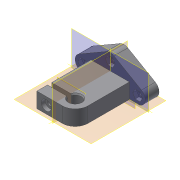
# Autodesk Inventor part: Cycl_soporteYfrenteDerecha
Saved by Autodesk Inventor 2015 SP2 (Build 190223200, 223)
## iProperties
Created: 2015-05-04
Material: Genérico
Document SubType Name: Modeling
Designer: E.Beroiz
Density: 1 g/cm^3
Appearance: Valor por defecto
Description: Cycl_soporteYfrenteDerecha
Author: E.Beroiz
Autodesk Inventor part; units mm, degrees
sketch "Boceto1" plane through (0, 0, 0) normal (0, 0, 1) x (1, 0, 0)
  line L0 (-13.875, 0) -> (13.875, 0)
  line L1 (13.875, 0) -> (13.875, -39.25)
  line L2 (13.875, -39.25) -> (-13.875, -39.25)
  line L3 (-13.875, -39.25) -> (-13.875, 0)
  point P0 (0, 0)
  point P1 (0, 0)
  dimension "d0" = 27.75
  dimension "d1" = 39.25
  constraints: 8 end point, 2 coincident, 2 parallel, 1 horizontal, 1 midpoint, 1 perpendicular
  measures "d0" distance of L1.end L2.end
  measures "d1" distance of L0.end L1.end
extrude "Extrusión1" add sketch "Boceto1" along normal blind 11
fillet "Empalme1" radius 9.25 1 edges at (13.875, -39.25, 5.5)
sketch "Boceto2" plane through (0, 0, 11) normal (0, 0, 1) x (1, 0, 0)
  arc A0 (4.625, -39.25) -> (13.875, -30) centre (4.625, -30) ccw projected
  line L0 (13.875, -30) -> (13.875, 0) projected
  line L1 (13.875, 0) -> (-13.875, 0) projected
  line L2 (-13.875, 0) -> (-13.875, -39.25) projected
  line L3 (-13.875, -39.25) -> (4.625, -39.25) projected
  line L4 (-13.875, 0) -> (-13.875, -39.25) projected
  line L5 (-13.875, -31.5) -> (0.4886, -31.5)
  line L6 (-13.875, -28.5) -> (0.4886, -28.5)
  arc A1 (0.4886, -31.5) -> (0.4886, -28.5) centre (4.625, -30) ccw
  point P0 (0, 0)
  dimension "d5" = 3
  dimension "d6" = 7.75
  dimension "d13" = 1.5
  dimension "d62" = 4.4
  dimension "d63" = 9.25
  constraints: 4 end point, 2 point on circle, 2 point on line, 1 centre point, 1 horizontal, 1 perpendicular
  measures "d5" distance between parallel lines of L6 L5
  measures "d6" distance between parallel lines of L3 L5
  measures "d13" distance from line of L5 A1.centre
  measures "d62" radius of A1
  measures "d63" distance from line of A0.centre L0
extrude "Extrusión2" cut sketch "Boceto2" against normal blind 11 contours L2 L6 A1 L5
sketch "Boceto3" plane through (0, 0, 0) normal (0, 1, 0) x (-1, 0, 0)
  line L0 (-19.875, 0) -> (19.875, 0)
  line L1 (22.6302, 10.2645) -> (2.7552, 21.7625)
  line L2 (-2.7552, 21.7625) -> (-22.6302, 10.2645)
  line L3 (13.875, 0) -> (-13.875, 0) projected
  arc A0 (-22.6302, 10.2645) -> (-19.875, 0) centre (-19.875, 5.502) ccw
  arc A1 (19.875, 0) -> (22.6302, 10.2645) centre (19.875, 5.502) ccw
  arc A2 (2.7552, 21.7625) -> (-2.7552, 21.7625) centre (0, 17) ccw
  point P0 (0, 0)
  point P1 (0, 23.3564)
  point P2 (0, 0)
  point P3 (0, 0)
  point P4 (0, 0)
  point P5 (0, 0)
  dimension "d21" = 30.05
  dimension "d23" = 39.75
  dimension "d25" = 17
  constraints: 6 end point, 6 point on circle, 6 tangent, 4 midpoint, 3 centre point, 2 equal radius, 2 point on line, 2 vertical alignment, 1 coincident, 1 equal length, 1 horizontal, 1 horizontal alignment
  measures "d21" angle of L0 L1
  measures "d23" distance of A1.centre A0.centre
  measures "d25" distance from line of L0 A2.centre
extrude "Extrusión3" add sketch "Boceto3" along normal blind 10
ref_plane "Plano de trabajo2" through (0, 7.2, 0) normal (0, 1, 0) x (1, 0, 0)
sketch "Boceto5" plane through (0, 7.2, 0) normal (0, 1, 0) x (1, 0, 0)
  line L0 (19.875, 0) -> (-19.875, 0) projected
  arc A0 (-19.875, 0) -> (-22.6302, -10.2645) centre (-19.875, -5.502) ccw projected
  line L1 (-22.6302, -10.2645) -> (-2.7552, -21.7625) projected
  arc A1 (-2.7552, -21.7625) -> (2.7552, -21.7625) centre (0, -17) ccw projected
  line L2 (2.7552, -21.7625) -> (22.6302, -10.2645) projected
  arc A2 (22.6302, -10.2645) -> (19.875, 0) centre (19.875, -5.502) ccw projected
  circle A3 centre (19.875, -5.502) radius 1.875
  circle A4 centre (0, -17) radius 1.875
  circle A5 centre (-19.875, -5.502) radius 1.875
  point P0 (0, 0)
  dimension "d33" = 3.75
  dimension "d34" = 3.75
  dimension "d35" = 3.75
  constraints: 3 centre point, 3 coincident
  measures "d33" diameter of A3
  measures "d34" diameter of A4
  measures "d35" diameter of A5
extrude "Extrusión5" cut sketch "Boceto5" along normal through all both and the other way through all contours A3 | A4 | A5
sketch "Boceto6" plane through (0, 0, 0) normal (0, -1, 0) x (1, 0, 0)
  circle A0 centre (0, 17) radius 1.875 projected
  circle A1 centre (19.875, 5.502) radius 1.875 projected
  circle A2 centre (-19.875, 5.502) radius 1.875 projected
  line L0 (13.875, 0) -> (13.875, 11) projected
  line L1 (19.875, 0) -> (13.875, 0) projected
  arc A3 (19.875, 0) -> (22.6302, 10.2645) centre (19.875, 5.502) ccw projected
  line L2 (2.7552, 21.7625) -> (22.6302, 10.2645) projected
  arc A4 (2.7552, 21.7625) -> (-2.7552, 21.7625) centre (0, 17) ccw projected
  line L3 (-22.6302, 10.2645) -> (-2.7552, 21.7625) projected
  arc A5 (-22.6302, 10.2645) -> (-19.875, 0) centre (-19.875, 5.502) ccw projected
  line L4 (-13.875, 0) -> (-19.875, 0) projected
  line L5 (-13.875, 0) -> (-13.875, 11) projected
  line L6 (13.875, 11) -> (-13.875, 11) projected
  line L7 (-18.0852, 8.602) -> (-16.2954, 5.502)
  line L8 (-16.2954, 5.502) -> (-18.0852, 2.402)
  line L9 (-18.0852, 2.402) -> (-21.6648, 2.402)
  line L10 (-21.6648, 2.402) -> (-23.4546, 5.502)
  line L11 (-23.4546, 5.502) -> (-21.6648, 8.602)
  line L12 (-21.6648, 8.602) -> (-18.0852, 8.602)
  line L13 (1.7898, 20.1) -> (3.5796, 17)
  line L14 (3.5796, 17) -> (1.7898, 13.9)
  line L15 (1.7898, 13.9) -> (-1.7898, 13.9)
  line L16 (-1.7898, 13.9) -> (-3.5796, 17)
  line L17 (-3.5796, 17) -> (-1.7898, 20.1)
  line L18 (-1.7898, 20.1) -> (1.7898, 20.1)
  line L19 (18.0852, 8.602) -> (21.6648, 8.602)
  line L20 (21.6648, 8.602) -> (23.4546, 5.502)
  line L21 (23.4546, 5.502) -> (21.6648, 2.402)
  line L22 (21.6648, 2.402) -> (18.0852, 2.402)
  line L23 (18.0852, 2.402) -> (16.2954, 5.502)
  line L24 (16.2954, 5.502) -> (18.0852, 8.602)
  point P0 (0, 0)
  dimension "d38" = 6.2
  dimension "d39" = 6.2
  dimension "d40" = 6.2
  constraints: 36 end point, 3 coincident, 3 horizontal, 39 other
  measures "d38" distance between parallel lines of L15 L18
  measures "d39" distance between parallel lines of L22 L19
  measures "d40" distance between parallel lines of L9 L12
extrude "Extrusión6" cut sketch "Boceto6" against normal blind 2.8 contours L7 L8 L9 L10 L11 L12 | L13 L14 L15 L16 L17 L18 | L19 L20 L21 L22 L23 L24
sketch "Boceto7" plane through (-13.875, -39.25, 0) normal (0, -1, 0) x (1, 0, 0)
  circle A0 centre (6.8, 5.5) radius 3.6
  line L0 (18.5, 0) -> (0, 0) projected
  line L1 (0, 0) -> (0, 11) projected
  point P0 (13.875, 0)
  dimension "d43" = 7.2
  dimension "d44" = 5.5
  dimension "d45" = 6.8
  constraints: 1 centre point
  measures "d43" diameter of A0
  measures "d44" distance from line of L0 A0.centre
  measures "d45" distance from line of L1 A0.centre
extrude "Extrusión7" cut sketch "Boceto7" against normal blind 2.8
sketch "Boceto8" plane through (-7.075, -36.45, 5.5) normal (0, -1, 0) x (1, 0, 0)
  circle A0 centre (0, 0) radius 3.6 projected
  circle A1 centre (0, 0) radius 1.875
  point P0 (7.075, -5.5)
  dimension "d48" = 3.75
  constraints: 1 centre point, 1 coincident
  measures "d48" diameter of A1
extrude "Extrusión8" cut sketch "Boceto8" against normal blind 26.4 contours A1
ref_plane "Plano de trabajo3" through (-13.875, -23.54, 0) normal (0, -1, 0) x (1, 0, 0)
sketch "Boceto9" plane through (-13.875, -23.54, 0) normal (0, -1, 0) x (1, 0, 0)
  circle A0 centre (6.8, 5.5) radius 1.875 projected
  line L0 (27.75, 11) -> (0, 11) projected
  line L1 (0, 0) -> (0, 11) projected
  line L2 (-21.6528, 0) -> (49.4028, 0) projected
  line L3 (8.7816, 8.5126) -> (10.3998, 5.2902)
  line L4 (10.3998, 5.2902) -> (8.4182, 2.2776)
  line L5 (8.7816, 8.5126) -> (0, 8.5126)
  line L6 (8.4182, 2.2776) -> (0, 2.2776)
  point P0 (13.875, 0)
  dimension "d53" = 120
  dimension "d56" = 6.235
  dimension "d57" = 8.7816
  constraints: 8 end point, 2 perpendicular, 2 point on line, 1 coincident, 4 other
  measures "d53" angle of L4 L3
  measures "d56" distance between parallel lines of L6 L5
  measures "d57" distance of L5.end L3.start
extrude "Extrusión9" cut sketch "Boceto9" along normal mid plane 2.8
sketch "Boceto10" plane through (0, 0, 0) normal (0, 0, -1) x (-1, 0, 0)
  line L0 (-6.6202, -3.2438) -> (-7.3905, -2.9152) construction
  line L1 (-8.0553, -2.0944) -> (-6.2205, -2.0944) construction
  line L2 (-7.3905, -2.9152) -> (-8.2942, -2.6479) construction
  line L3 (-8.8708, -2.1991) -> (-8.0553, -2.0944) construction
  line L4 (-8.2942, -2.6479) -> (-9.3576, -2.433) construction
  line L5 (-9.521, -2.3562) -> (-8.8708, -2.1991) construction
  line L6 (-9.5623, -2.392) -> (-9.521, -2.3562) construction
  line L7 (-9.3576, -2.433) -> (-9.5623, -2.392) construction
  arc A0 (-6.6202, -3.2438) -> (-9.5623, -2.392) centre (-11.1752, -13.4701) ccw
  line L8 (-4.1904, -17.1175) -> (-4.9646, -16.4122) construction
  line L9 (-2.3638, -18.1479) -> (-2.8515, -17.944) construction
  line L10 (-2.2067, -18.1953) -> (-2.372, -18.0796) construction
  line L11 (-6.5651, -9.2139) -> (-6.3061, -8.5334) construction
  line L12 (-6.7552, -9.9275) -> (-6.5651, -9.2139) construction
  line L13 (-6.8626, -10.619) -> (-6.7552, -9.9275) construction
  line L14 (-6.3061, -8.5334) -> (-5.981, -7.886) construction
  line L15 (-5.981, -7.886) -> (-5.5953, -7.2826) construction
  line L16 (-5.5953, -7.2826) -> (-5.1545, -6.7234) construction
  line L17 (-4.6724, -6.0787) -> (-4.733, -5.5552) construction
  line L18 (-4.6614, -6.2109) -> (-4.6724, -6.0787) construction
  line L19 (-5.1545, -6.7234) -> (-4.6614, -6.2109) construction
  arc A1 (-4.6614, -6.2109) -> (-6.8626, -10.619) centre (0.1756, -11.3801) ccw
  line L20 (-6.8489, -12.3602) -> (-1.9257, -12.3602)
  line L21 (-2.0248, -10.619) -> (-6.8626, -10.619) construction
  line L22 (-2.0248, -10.619) -> (-6.8626, -10.619)
  line L23 (-3.3198, -17.7016) -> (-3.7661, -17.4261) construction
  line L24 (-3.7661, -17.4261) -> (-4.1904, -17.1175) construction
  line L25 (-2.8515, -17.944) -> (-3.3198, -17.7016) construction
  line L26 (-4.9646, -16.4122) -> (-5.6285, -15.594) construction
  line L27 (-5.6285, -15.594) -> (-5.9123, -15.1504) construction
  line L28 (-5.9123, -15.1504) -> (-6.1658, -14.682) construction
  arc A2 (-6.8489, -12.3602) -> (-2.3638, -18.1479) centre (0.1619, -11.559) ccw
  line L29 (-6.1658, -14.682) -> (-6.3834, -14.1944) construction
  line L30 (-0.5371, -13.4071) -> (-0.1239, -13.4484) construction
  line L31 (-0.9228, -13.2858) -> (-0.5371, -13.4071) construction
  line L32 (-1.2727, -13.0985) -> (-0.9228, -13.2858) construction
  line L33 (-6.8489, -12.3602) -> (-1.9257, -12.3602) construction
  line L34 (-6.3834, -14.1944) -> (-6.568, -13.6847) construction
  line L35 (-6.568, -13.6847) -> (-6.7112, -13.1613) construction
  line L36 (-6.7112, -13.1613) -> (-6.8268, -12.553) construction
  line L37 (-6.8268, -12.553) -> (-6.8489, -12.3602) construction
  line L38 (1.5815, -12.542) -> (1.7688, -12.1921) construction
  line L39 (1.025, -13.0985) -> (1.328, -12.845) construction
  line L40 (0.6751, -13.2858) -> (1.025, -13.0985) construction
  line L41 (0.2894, -13.4071) -> (0.6751, -13.2858) construction
  line L42 (-0.1239, -13.4484) -> (0.2894, -13.4071) construction
  line L43 (1.328, -12.845) -> (1.5815, -12.542) construction
  line L44 (1.328, -9.9412) -> (1.025, -9.6905) construction
  line L45 (1.025, -9.6905) -> (0.6751, -9.5004) construction
  line L46 (1.7688, -10.5942) -> (1.5815, -10.2443) construction
  line L47 (1.5815, -10.2443) -> (1.328, -9.9412) construction
  line L48 (1.89, -10.9799) -> (1.7688, -10.5942) construction
  line L49 (0.6751, -9.5004) -> (0.2894, -9.382) construction
  line L50 (1.9314, -11.3931) -> (1.89, -10.9799) construction
  line L51 (0.2894, -9.382) -> (-0.1239, -9.3406) construction
  line L52 (-1.9257, -12.3602) -> (-1.8292, -12.542) construction
  line L53 (-1.8292, -12.542) -> (-1.5758, -12.845) construction
  line L54 (-1.5758, -12.845) -> (-1.2727, -13.0985) construction
  line L55 (1.89, -11.8064) -> (1.9314, -11.3931) construction
  line L56 (1.7688, -12.1921) -> (1.89, -11.8064) construction
  arc A3 (-1.9257, -12.3602) -> (-2.0248, -10.619) centre (-0.0805, -11.3816) ccw
  line L57 (-2.6748, -2.6372) -> (-1.5397, -2.9457) construction
  arc A4 (2.4908, -4.8109) -> (-9.5623, -2.392) centre (-6.7465, -19.6002) ccw
  line L58 (-3.8457, -2.3892) -> (-2.6748, -2.6372) construction
  line L59 (-5.9617, -3.6405) -> (-6.6202, -3.2438) construction
  line L60 (-5.5678, -3.9821) -> (-5.9617, -3.6405) construction
  line L61 (-6.2205, -2.0944) -> (-5.0331, -2.2074) construction
  line L62 (-5.2317, -4.3596) -> (-5.5678, -3.9821) construction
  line L63 (-5.0002, -4.7342) -> (-5.2317, -4.3596) construction
  arc A5 (-4.6614, -6.2109) -> (-6.6202, -3.2438) centre (-7.8027, -6.1546) ccw
  line L64 (-4.8377, -5.1199) -> (-5.0002, -4.7342) construction
  line L65 (-4.733, -5.5552) -> (-4.8377, -5.1199) construction
  line L66 (-5.0331, -2.2074) -> (-3.8457, -2.3892) construction
  line L67 (1.477, -4.1745) -> (2.2925, -4.6676) construction
  line L68 (0.5541, -3.7199) -> (1.477, -4.1745) construction
  line L69 (-0.457, -3.3094) -> (0.5541, -3.7199) construction
  line L70 (-1.5397, -2.9457) -> (-0.457, -3.3094) construction
  line L71 (2.2925, -4.6676) -> (2.4908, -4.8109) construction
  line L72 (4.7417, -16.6134) -> (4.7555, -16.7815) construction
  line L73 (5.2266, -16.1038) -> (4.7417, -16.6134) construction
  line L74 (6.0393, -14.9466) -> (5.6619, -15.5472) construction
  line L75 (2.4908, -4.8109) -> (2.9702, -5.0203) construction
  line L76 (2.9702, -5.0203) -> (3.4331, -5.2627) construction
  line L77 (3.4331, -5.2627) -> (4.2899, -5.8495) construction
  line L78 (4.2899, -5.8495) -> (5.0502, -6.5548) construction
  line L79 (5.0502, -6.5548) -> (5.7032, -7.3676) construction
  line L80 (5.7032, -7.3676) -> (6.2321, -8.2767) construction
  line L81 (6.2321, -8.2767) -> (6.447, -8.7616) construction
  arc A6 (4.7555, -16.7815) -> (2.4908, -4.8109) centre (-0.321, -11.5424) ccw
  line L82 (6.3589, -14.3047) -> (6.0393, -14.9466) construction
  line L83 (5.6619, -15.5472) -> (5.2266, -16.1038) construction
  line L84 (6.447, -8.7616) -> (6.6261, -9.2658) construction
  line L85 (4.8161, -17.305) -> (4.9235, -17.7402) construction
  line L86 (4.9235, -17.7402) -> (5.0861, -18.126) construction
  line L87 (4.7555, -16.7815) -> (4.8161, -17.305) construction
  line L88 (5.0861, -18.126) -> (5.3175, -18.5006) construction
  line L89 (5.3175, -18.5006) -> (5.6536, -18.8781) construction
  line L90 (5.6536, -18.8781) -> (6.0986, -19.2458) construction
  line L91 (6.2225, -20.7819) -> (5.0379, -20.669) construction
  arc A7 (4.7555, -16.7815) -> (6.757, -19.6425) centre (8.0368, -16.6165) ccw
  line L92 (6.0986, -19.2458) -> (6.757, -19.6425) construction
  line L93 (7.1537, -20.7985) -> (6.2225, -20.7819) construction
  line L94 (6.757, -19.6425) -> (7.4717, -19.9448) construction
  line L95 (6.6261, -9.2658) -> (6.7694, -9.7837) construction
  line L96 (6.7694, -9.7837) -> (6.8713, -10.321) construction
  line L97 (6.9347, -10.8692) -> (6.9567, -11.4312) construction
  line L98 (6.9567, -11.4312) -> (6.9181, -12.1889) construction
  line L99 (6.9181, -12.1889) -> (6.8024, -12.9245) construction
  line L100 (6.8024, -12.9245) -> (6.6151, -13.6297) construction
  line L101 (6.6151, -13.6297) -> (6.3589, -14.3047) construction
  line L102 (6.8713, -10.321) -> (6.9347, -10.8692) construction
  line L103 (7.4717, -19.9448) -> (8.3753, -20.212) construction
  arc A8 (6.757, -19.6425) -> (9.6454, -20.4682) centre (11.2767, -9.2971) ccw
  line L104 (8.3753, -20.212) -> (9.4388, -20.4269) construction
  line L105 (9.4388, -20.4269) -> (9.6454, -20.4682) construction
  line L106 (8.1384, -20.7658) -> (7.2348, -20.785) construction
  line L107 (8.9539, -20.6611) -> (8.1384, -20.7658) construction
  line L108 (9.6041, -20.504) -> (8.9539, -20.6611) construction
  line L109 (9.6454, -20.4682) -> (9.6041, -20.504) construction
  line L110 (5.0379, -20.669) -> (3.8505, -20.4872) construction
  line L111 (3.8505, -20.4872) -> (2.6796, -20.2392) construction
  arc A9 (-2.3638, -18.1479) -> (9.6454, -20.4682) centre (6.7458, -3.2373) ccw
  line L112 (2.6796, -20.2392) -> (1.5445, -19.9306) construction
  line L113 (0.5428, -19.5535) -> (-0.4683, -19.143) construction
  line L114 (-0.4683, -19.143) -> (-1.3912, -18.6885) construction
  line L115 (-1.3912, -18.6885) -> (-2.2067, -18.1953) construction
  line L116 (1.6255, -19.9172) -> (0.5428, -19.5535) construction
  line L117 (-2.0166, -10.5942) -> (-2.0248, -10.619) construction
  line L118 (-1.8292, -10.2443) -> (-2.0166, -10.5942) construction
  line L119 (-1.5758, -9.9412) -> (-1.8292, -10.2443) construction
  line L120 (-1.2727, -9.6905) -> (-1.5758, -9.9412) construction
  line L121 (-0.9228, -9.5004) -> (-1.2727, -9.6905) construction
  line L122 (-0.5371, -9.382) -> (-0.9228, -9.5004) construction
  line L123 (-0.1239, -9.3406) -> (-0.5371, -9.382) construction
  point P0 (0, 0)
  constraints: 248 end point, 24 point on circle, 10 centre point
extrude "Extrusión10" cut sketch "Boceto10" against normal blind 2
sketch "Boceto11" plane through (0, 2.8, 0) normal (0, -1, 0) x (1, 0, 0)
  point P0 (0, 0)
chamfer "Chamfer1" distance 1 angle 30 2 edges at (9.025, -30, 0) (9.025, -30, 11) measured on face at (8.0232, -32.795, 3.6667)
